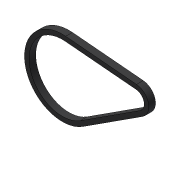
# Autodesk Inventor part: CHAIN
Saved by Autodesk Inventor 2022.5 (Build 265521000, 521)
## iProperties
Created: 2023-02-21
Part Number: CHAIN
Material: 일반
Description: 3
Document SubType Name: Modeling
Designer: 박성규
Density: 1 g/cm^3
Appearance: 일반
User Status: 1
DETAIL: Coveryor Assembly
M/C TITLE: MEa/NEa차종 시트조립라인
MAKER: HANKOOK CHAIN
SPECIFICATION: TA20221101-CV200000-015
DocNumber: 221118_Standard_v1
Folder: .\
VDS_Category: 엔지니어링
Detail Description: Purchased products
Title: RS35x61LINK
Author: 박성규
Revision Number: B
Autodesk Inventor part; units mm, degrees
ref_plane "YZ Plane" through (0, 0, 0) normal (1, 0, 0) x (0, 1, 0)
ref_plane "XZ Plane" through (0, 0, 0) normal (0, 1, 0) x (-1, 0, 0)
ref_plane "XY Plane" through (0, 0, 0) normal (0, 0, 1) x (1, 0, 0)
sketch "스케치9" plane through (0, 0, 0) normal (0, 0, 1) x (1, 0, 0)
  circle A0 centre (0, 0) radius 68.275 construction
  circle A1 centre (140, 34.65) radius 21.405 construction
  line L0 (6.0254, 68.0086) -> (141.889, 55.9715)
  line L1 (151.6159, 16.671) -> (37.0509, -57.3472)
  arc A2 (6.0254, 68.0086) -> (37.0509, -57.3472) centre (0, 0) ccw
  arc A3 (151.6159, 16.671) -> (141.889, 55.9715) centre (140, 34.65) ccw
  line L2 (0, 0) -> (585.5568, 0) construction
  dimension "d40" = 42.81
  dimension "d41" = 136.55
  dimension "d43" = 34.65
  dimension "d53" = 140
  dimension "d54" = 259.689
  dimension "d55" = 136.3958
  dimension "d56" = 136.3958
  dimension "d57" = 53.0761
  dimension "d58" = 585.5568
  constraints: 8 point on circle, 6 end point, 4 centre point, 4 tangent, 3 coincident, 1 horizontal
  measures "d40" diameter of A1
  measures "d41" diameter of A0
  measures "d43" vertical distance of A1.centre point (0, 0)
  measures "d53" horizontal distance of A1.centre point (0, 0)
  measures "d55" distance of L0.start L0.end
  measures "d56" distance of L1.start L1.end
  measures "d58" distance of L2.start L2.end
sketch "스케치10" plane through (0, 0, 0) normal (1, 0, 0) x (0, 1, 0)
  line L0 (72.675, 6.4) -> (63.875, 6.4)
  line L1 (63.875, 6.4) -> (63.875, -6.4)
  line L2 (63.875, -6.4) -> (72.675, -6.4)
  line L3 (72.675, -6.4) -> (72.675, 6.4)
  line L4 (72.675, 6.4) -> (63.875, -6.4) construction
  line L5 (63.875, 6.4) -> (72.675, -6.4) construction
  point P0 (0, 0)
  point P1 (68.275, 0)
  point P2 (68.275, 0)
  dimension "d44" = 12.8
  dimension "d45" = 8.8
  dimension "d46" = 68.275
  constraints: 12 end point, 3 midpoint, 2 parallel, 1 horizontal, 1 horizontal alignment, 1 perpendicular
  measures "d44" distance of L2.end L0.start
  measures "d45" distance of L1.end L2.end
  measures "d46" distance of point (0, 0) point (68.275, 0)
sweep "스윕1" add profiles "스케치10" path "스케치9" path curves L0 A3 L1 A2
equation "\"d58\" = d54 + d55 + d56 + d57"
